1.3mm_closer1 (Autodesk Fusion 360 design; units mm, degrees)
Autodesk Fusion 360 part; units mm, degrees
sketch "Sketch1" plane through (0, 0, 0) normal (0, 1, 0) x (1, 0, 0)
  line L0 (0, 0) -> (0, -10)
  line L1 (0, -10) -> (-11.5, -10)
  line L2 (-11.5, -10) -> (-11.5, -7.6)
  line L3 (-11.5, -7.6) -> (-6.5, -7.6)
  line L4 (-6.5, -7.6) -> (-6.5, -0.8)
  line L5 (-6.5, -0.8) -> (-3, -0.8)
  line L6 (-3, -0.8) -> (-3, 0)
  line L7 (-3, 0) -> (0, 0)
  dimension "d1" = 10
  dimension "d2" = 3
  dimension "d4" = 7.6
  dimension "d5" = 5
  dimension "d7" = 0.8
  dimension "d8" = 3.5
  constraint coincident L0.start L7.end
  constraint vertical L0
  constraint perpendicular L0 L1
  constraint perpendicular L1 L2
  constraint perpendicular L0 L3
  constraint perpendicular L1 L4
  constraint perpendicular L4 L5
  constraint perpendicular L1 L6
  constraint perpendicular L0 L7
  measures "d1" distance of L0.start L0.end
  measures "d2" distance of L6.end L0.start
  measures "d4" distance of L0.start L3
  measures "d5" distance of L2.end L3.end
  measures "d7" distance of L0.start L5
  measures "d8" distance of L4.end L5.end
revolve "Revolve1" add sketch "Sketch1" angle 360 about axis through (1.75, 0, 0) along (1, 0, 0)
sketch "Sketch3" plane through (0, 0, 0) normal (1, 0, 0) x (0, 1, 0)
  line L0 (7.0397, 1.6829) -> (-6.9599, 1.688) construction
  line L1 (-6.9599, 1.688) -> (-6.9635, -8.3124) construction
  line L2 (-6.9635, -8.3124) -> (7.0361, -8.3175) construction
  line L3 (7.0361, -8.3175) -> (7.0397, 1.6829) construction
  circle A0 centre (0, 0) radius 10
  line L4 (7.0397, 1.6829) -> (-6.9599, 1.688) construction
  line L5 (-6.9599, 1.688) -> (-6.9635, -8.3124) construction
  line L6 (-6.9635, -8.3124) -> (7.0361, -8.3175) construction
  line L7 (7.0361, -8.3175) -> (7.0397, 1.6829) construction
  line L8 (7.0397, 7.6829) -> (-6.9599, 7.688) construction
  line L9 (-6.9599, 7.688) -> (-6.9635, -2.3124) construction
  line L10 (-6.9635, -2.3124) -> (7.0361, -2.3175) construction
  line L11 (7.0361, -2.3175) -> (7.0397, 7.6829) construction
  dimension "d13" = 3
  dimension "d20" = 3
  dimension "d21" = 5
  text T0 "1.3 mm" font "Arial" height 3 align centre middle in box 13.9996 x 10.0004 at (7.0397, 1.6829) x (-1, 0.00036) y (-0.00036, -1) spacing 1
  text T1 "A" font "Arial" height 5 align centre middle in box 13.9996 x 10.0004 at (7.0397, 7.6829) x (-1, 0.00036) y (-0.00036, -1) spacing 1
emboss "Emboss1" depth 0.4 profiles "Sketch3" section 1 text T0 T1 onto face at (0, 1.6236, 1.9302)
fillet "Fillet2" radius 0.5 1 edges at (-6.5, -0.2893, -0.7459)
fillet "Fillet1" radius 0.5 3 edges at (-11.5, -3.6162, -9.3233) (-11.5, -2.7483, -7.0857) (0, -3.6162, -9.3233)
equation "d7 = 1.6 mm / 2"
